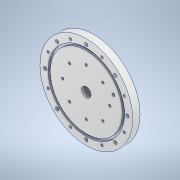
# Autodesk Inventor part: Base_Bowl_Glovebox
Saved by Autodesk Inventor 2021 (Build 250183000, 183)
## iProperties
Created: 2021-02-09
Part Number: Base_Bowl_Glovebox
Material: Aluminum 6061
Document SubType Name: Modeling
Designer: Timo
Density: 2.7 g/cm^3
Appearance: Aluminum - Flat
Author: Timo
Autodesk Inventor part; units mm, degrees
ref_plane "YZ Plane" through (0, 0, 0) normal (1, 0, 0) x (0, 1, 0)
ref_plane "XZ Plane" through (0, 0, 0) normal (0, 1, 0) x (-1, 0, 0)
ref_plane "XY Plane" through (0, 0, 0) normal (0, 0, 1) x (1, 0, 0)
sketch "Sketch1" plane through (0, 0, 0) normal (0, 0, 1) x (1, 0, 0)
  circle A0 centre (0, 0) radius 63
  dimension "d0" = 126
  constraints: 1 centre point, 1 coincident
  measures "d0" diameter of A0
extrude "Extrusion1" add sketch "Sketch1" along normal blind 10
sketch "Sketch3" plane through (0, 0, 10) normal (0, 0, 1) x (1, 0, 0)
  circle A0 centre (0, 0) radius 52
  circle A1 centre (0, 0) radius 49
  dimension "d11" = 3
  dimension "d35" = 98
  constraints: 2 centre point, 1 coincident
  measures "d11" radial gap between concentric circles of A0 A1
  measures "d35" diameter of A1
extrude "Extrusion3" cut sketch "Sketch3" against normal blind 2.5
sketch "Sketch2" plane through (0, 0, 10) normal (0, 0, 1) x (1, 0, 0)
  circle A0 centre (0, 0) radius 56 construction
  circle A1 centre (0, 56) radius 2.2
  line L0 (0, -88.2) -> (0, 88.2) projected
  dimension "d3" = 112
  dimension "d4" = 4.4
  constraints: 1 centre point, 1 coincident, 1 point on line, 1 vertical alignment, 2 other
  measures "d4" diameter of A1
extrude "Extrusion2" cut sketch "Sketch2" against normal blind 10
pattern_circular "Circular Pattern1" count 8 over 360 about axis through (0, 0, -10) along (0, 0, 1) of "Extrusion2"
sketch "Sketch4" plane through (0, 0, 10) normal (0, 0, 1) x (1, 0, 0)
  circle A0 centre (0, 0) radius 32 construction
  line L0 (0, -88.2) -> (0, 88.2) construction
  point P0 (0, 32)
  dimension "d14" = 64
  constraints: 1 coincident, 1 point on line, 1 vertical alignment, 2 other
hole "Hole1" at (0, 32, 10) direction (0, 0, -1) diameter 3.242 depth 8 thread size "M4x0.7" class "6H" standard "ANSI Metric M Profile"
pattern_circular "Circular Pattern2" count 8 over 360 about axis through (0, 0, -10) along (0, 0, 1) of "Hole1"
sketch "Sketch5" plane through (0, 0, 10) normal (0, 0, 1) x (1, 0, 0)
  circle A0 centre (36.9552, 15.3073) radius 2
  circle A1 centre (22.6274, 22.6274) radius 1.621 construction
  line L0 (22.6274, 22.6274) -> (0, 0) construction
  line L1 (0, 0) -> (36.9552, 15.3073) construction
  line L2 (-88.2, 0) -> (88.2, 0) construction
  circle A2 centre (0, 0) radius 42 construction
  dimension "d25" = 4
  dimension "d26" = 45
  dimension "d27" = 22.5
  dimension "d29" = 84
  constraints: 4 end point, 2 centre point, 1 coincident, 1 tangent
  measures "d25" diameter of A0
  measures "d26" angle of L2 L0
  measures "d27" angle of L2 L1
  measures "d29" diameter of A2
extrude "Extrusion4" cut sketch "Sketch5" against normal through all
sketch "Sketch6" plane through (0, 0, 10) normal (0, 0, 1) x (1, 0, 0)
  circle A0 centre (0, 0) radius 6.5
  dimension "d32" = 13
  constraints: 1 centre point, 1 coincident
  measures "d32" diameter of A0
extrude "Extrusion5" cut sketch "Sketch6" against normal through all
sketch "Sketch7" plane through (0, 0, 10) normal (0, 0, 1) x (1, 0, 0)
  circle A0 centre (0, 56) radius 2.2 construction
  circle A1 centre (0, 0) radius 56 construction
  line L0 (-21.4303, 51.7373) -> (0, 0) construction
  line L1 (0, 0) -> (0, 56) construction
  circle A2 centre (-39.598, 39.598) radius 2.2 construction
  line L2 (-39.598, 39.598) -> (0, 0) construction
  dimension "d36" = 45
  dimension "d37" = 22.5
  constraints: 6 end point, 2 point on circle, 1 centre point, 1 coincident, 1 vertical
  measures "d36" angle of L1 L2
  measures "d37" angle of L1 L0
hole "Hole2" at (-21.4303, 51.7373, 10) direction (0, 0, -1) diameter 3.242 end through all thread size "M4x0.7" class "6H" standard "ANSI Metric M Profile"
pattern_circular "Circular Pattern3" count 8 over 360 about axis through (0, 0, -10) along (0, 0, 1) of "Hole2"
equation "\"d27\" = 0.5 * d26"
equation "\"d37\" = 0.5 * d36"
body "Solid1"
